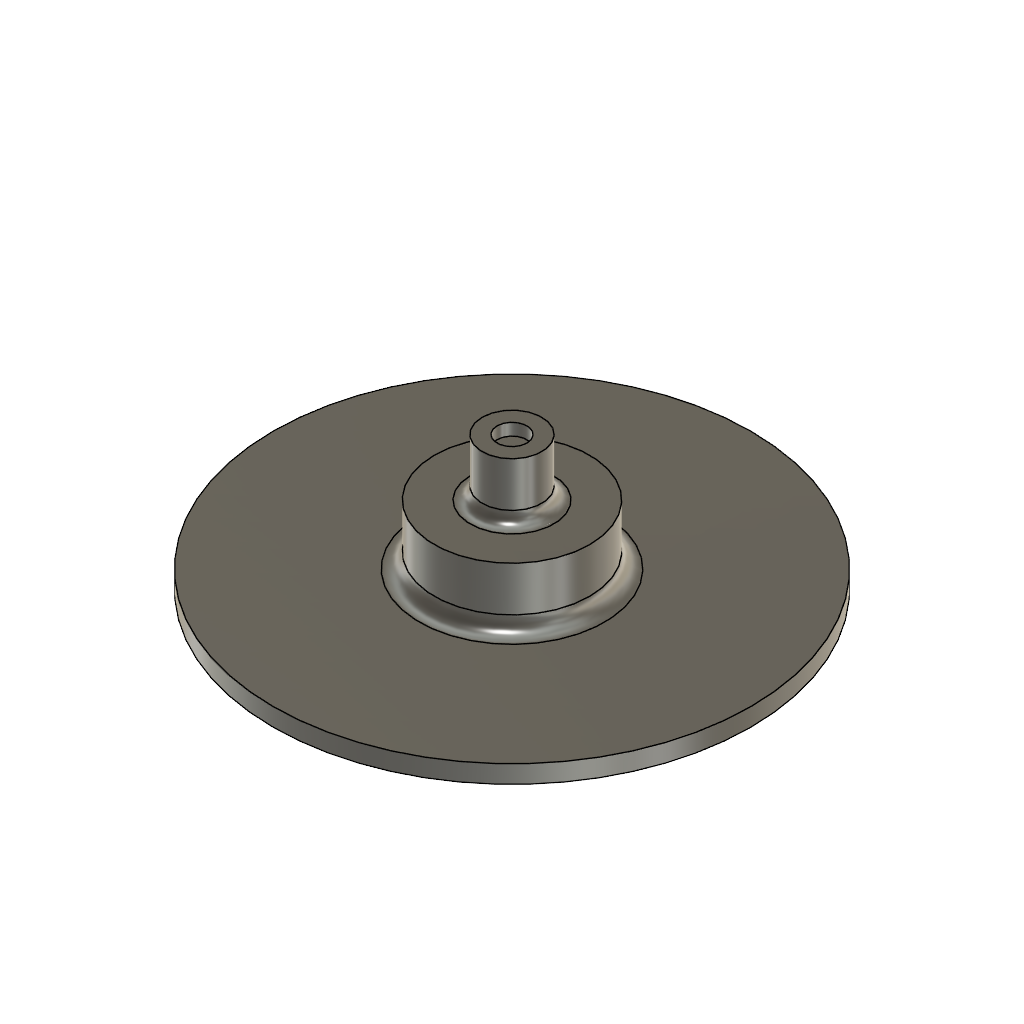
bearing_holder (Autodesk Fusion 360 design; units mm, degrees)
part number: 2026-09-09-05-31-22-504
Autodesk Fusion 360 part; units mm, degrees
sketch "Sketch1" plane through (0, 0, 0) normal (0, 0, 1) x (1, 0, 0)
  circle A0 centre (0, 0) radius 2.5
  circle A1 centre (0, 0) radius 5
  dimension "d1" = 5
  dimension "d2" = 10
  constraint coincident A0.centre A1.centre
  measures "d1" diameter of A0
  measures "d2" diameter of A1
extrude "Extrude1" add sketch "Sketch1" along normal blind 2
extrude "Extrude2" add sketch "Sketch1" against normal blind 5.5 contours A0 | A1
sketch "Sketch2" plane through (0, 0, -5.5) normal (0, 0, -1) x (1, 0, 0)
  circle A0 centre (0, 0) radius 5
  circle A1 centre (0, 0) radius 13
  dimension "d7" = 26
  constraint coincident A0.centre A1.centre
  measures "d7" diameter of A1
extrude "Extrude3" add sketch "Sketch2" along normal blind 5 contours A0 | A1
extrude "Extrude4" cut 1 faces at (10.2663, 0.8943, -5.5) along direction (0, 0, -1) blind 2
fillet "Fillet1" radius 2 1 edges at (-4.6616, -1.8081, -7.5)
extrude "Extrude5" add 1 faces at (2.1667, -3.7528, -10.5) along direction (0, 0, -1) blind 5.5
extrude "Extrude6" add 1 faces at (2.1667, -3.7528, -16) along direction (0, 0, -1) blind 1.5
sketch "Sketch3" plane through (0, 0, -17.5) normal (0, 0, -1) x (1, 0, 0)
  circle A0 centre (0, 0) radius 13
  circle A1 centre (0, 0) radius 40
  dimension "d18" = 80
  constraint coincident A0.centre A1.centre
  measures "d18" diameter of A1
extrude "Extrude7" add sketch "Sketch3" along normal blind 3 contours A0 | A1
fillet "Fillet2" radius 2.5 1 edges at (-12.1203, 4.701, -17.5)
